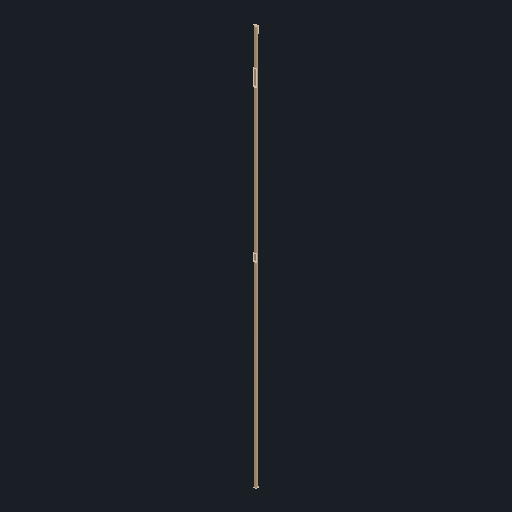
# Autodesk Inventor part: Rotating Rod 370mm
Saved by Autodesk Inventor 2027.1 (Build 311270010, 270A)
## iProperties
Created: 2025-09-16
Material: Stainless Steel
Document SubType Name: Modeling
Designer: SD
Density: 8 g/cm^3
Appearance: Brindle
Mass: 22.4035 g
Surface Area: 34.7152 cm^2
Volume: 2.52462 cm^3
Project: Automatic Tea Steeping mechanism
Part Number: Rotating Rod 370mm
Length: 370.000 mm
BOM-Mass: 0.02240
BOM-Area: 0.003
Diameter: 3.000 mm
Procurement: Fabricate - 1st round
Build Stage: 1
Preferred Material: 303 Stainless Steel
Author: SD
Title: Rotating Rod 370mm
Autodesk Inventor part; units mm, degrees
ref_plane "YZ Plane" through (0, 0, 0) normal (1, 0, 0) x (0, 1, 0)
ref_plane "XZ Plane" through (0, 0, 0) normal (0, 1, 0) x (-1, 0, 0)
ref_plane "XY Plane" through (0, 0, 0) normal (0, 0, 1) x (1, 0, 0)
sketch "Sketch4" plane through (0, 0, 0) normal (0, 1, 0) x (-1, 0, 0)
  circle A0 centre (0, 0) radius 1.5
  constraints: 1 centre point, 1 coincident, 1 other
extrude "Extrusion2" add sketch "Sketch4" along normal mid plane 370
sketch "Sketch13" plane through (0, 0, 0) normal (1, 0, 0) x (0, 1, 0)
  line L0 (185.7937, -0.5) -> (178, -0.5)
  line L1 (178, -0.5) -> (178, -2.4686)
  line L2 (178, -2.4686) -> (185.7937, -2.4686)
  line L3 (185.7937, -2.4686) -> (185.7937, -0.5)
  line L4 (-185, -1.5) -> (185, -1.5) projected
  line L5 (185, -1.5) -> (185, 1.5) projected
  line L6 (151, 2.5026) -> (136, 2.5026)
  line L7 (136, 2.5026) -> (136, 0.5)
  line L8 (136, 0.5) -> (151, 0.5)
  line L9 (151, 0.5) -> (151, 2.5026)
  line L10 (-185, 1.5) -> (185, 1.5) projected
  line L11 (-185, 1.5) -> (-185, -1.5) projected
  line L12 (3, 4.5) -> (-4, 4.5)
  line L13 (-4, 4.5) -> (-4, 0.5)
  line L14 (-4, 0.5) -> (3, 0.5)
  line L15 (3, 0.5) -> (3, 4.5)
  point P0 (0, 0)
  point P1 (151, 1.5)
  point P2 (136, 1.5)
  point P3 (185, -0.5)
  point P4 (178, -1.5)
  dimension "d89" = 1
  dimension "d90" = 7
  dimension "d91" = 1
  dimension "d92" = 15
  dimension "d96" = 34
  dimension "d97" = 1
  dimension "d98" = 7
  dimension "d99" = 182
  constraints: 24 end point, 6 parallel, 3 horizontal, 3 perpendicular
  measures "d89" distance between parallel lines of L4 L0
  measures "d90" distance between parallel lines of L1 L5
  measures "d91" distance between parallel lines of L8 L10
  measures "d92" distance of L6.start L6.end
  measures "d96" distance between parallel lines of L5 L9
  measures "d97" distance between parallel lines of L14 L10
  measures "d98" distance of L12.start L12.end
  measures "d99" distance between parallel lines of L5 L15
extrude "Extrusion9" cut sketch "Sketch13" against normal through all both and the other way through all contours L5 L4 L1 L0 | L9 L8 L7 L10 | L15 L14 L13 L10 | L10 L13 L12 L15
body "Solid2"
